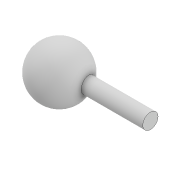
# Autodesk Inventor part: Input_Shaft
Saved by Autodesk Inventor 2022 (Build 260153000, 153)
## iProperties
Created: 2023-10-11
Part Number: Input_Shaft
Material: 一般
Document SubType Name: Modeling
Designer: JOU
Density: 1 g/cm^3
Appearance: 預設
Author: JOU
Autodesk Inventor part; units mm, degrees
ref_plane "YZ Plane" through (0, 0, 0) normal (1, 0, 0) x (0, 1, 0)
ref_plane "XZ Plane" through (0, 0, 0) normal (0, 1, 0) x (-1, 0, 0)
ref_plane "XY Plane" through (0, 0, 0) normal (0, 0, 1) x (1, 0, 0)
sketch "草圖1" plane through (0, 0, 0) normal (0, 0, 1) x (1, 0, 0)
  circle A0 centre (0, 0) radius 15
  line L0 (13.3309, -6.8766) -> (-13.3309, 6.8766)
  dimension "d0" = 30
  constraints: 2 end point, 2 point on circle, 1 centre point, 1 coincident, 1 midpoint
  measures "d0" diameter of A0
revolve "迴轉1" add sketch "草圖1" angle 360 about axis through (13.3309, -6.8766, 0) along (-0.8887264, 0.4584381, 0) picked at (5.5976, 4.8304) contours A0 L0
sketch "草圖2" plane through (0, 0, 0) normal (1, 0, 0) x (0, 1, 0)
  circle A0 centre (0, -2) radius 4.3537
  point P0 (0, 0)
  dimension "d2" = 2
  constraints: 1 centre point
  measures "d2" distance of point (0, 0) A0.centre
extrude "擠出1" add sketch "草圖2" along normal blind 50
